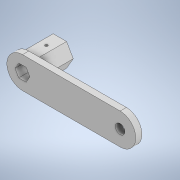
# Autodesk Inventor part: Acople_TransPot
Saved by Autodesk Inventor 2022 (Build 260153000, 153)
## iProperties
Created: 2022-02-22
Part Number: Acople_TransPot
Material: Generic
Document SubType Name: Modeling
Designer: katha
Density: 1 g/cm^3
Appearance: Default
Author: katha
Autodesk Inventor part; units mm, degrees
ref_plane "YZ Plane" through (0, 0, 0) normal (1, 0, 0) x (0, 1, 0)
ref_plane "XZ Plane" through (0, 0, 0) normal (0, 1, 0) x (-1, 0, 0)
ref_plane "Work Plane4" through (0, 0, 3) normal (0, 0, 1) x (1, 0, 0)
sketch "Sketch3" plane through (0, 0, 3) normal (0, 0, 1) x (1, 0, 0)
  circle A0 centre (47, 0) radius 2.3
  circle A1 centre (0, 0) radius 7.5 projected
  circle A2 centre (47, 0) radius 7.5
  line L0 (0, -7.5) -> (47, -7.5)
  line L1 (47, 0) -> (12.3969, 0) construction
  line L2 (0, 7.5) -> (47, 7.5)
  point P0 (0, 0)
  dimension "d13" = 15
  dimension "d5" = 4.6
  dimension "d14" = 47
  constraints: 6 end point, 3 horizontal, 2 symmetric about line, 1 centre point, 1 coincident, 5 other
  measures "d5" diameter of A0
  measures "d14" distance of L0.start L0.end
extrude "Extrusion5" add sketch "Sketch3" along normal blind 3
sketch "Sketch6" plane through (0, 0, 3) normal (0, 0, -1) x (-1, 0, 0)
  arc A0 (0, -7.5) -> (0, 7.5) centre (0, 0) ccw projected
  line L0 (0, 0) -> (3.1, 0) construction
  line L1 (0, 0) -> (1.55, 2.6847) construction
  line L2 (0, 0) -> (-1.55, 2.6847) construction
  line L3 (0, 0) -> (-3.1, 0) construction
  line L4 (0, 0) -> (-1.55, -2.6847) construction
  line L5 (0, 0) -> (1.55, -2.6847) construction
  line L6 (-1.55, 2.6847) -> (1.55, 2.6847) construction
  line L7 (1.55, 2.6847) -> (3.1, 0) construction
  line L8 (3.1, 0) -> (1.55, -2.6847) construction
  line L9 (1.55, -2.6847) -> (-1.55, -2.6847) construction
  line L10 (-1.55, -2.6847) -> (-3.1, 0) construction
  line L11 (-3.1, 0) -> (-1.55, 2.6847) construction
  line L12 (3.5619, 0) -> (1.7809, 3.0847)
  line L13 (1.7809, 3.0847) -> (-1.7809, 3.0847)
  line L14 (-1.7809, 3.0847) -> (-3.5619, 0)
  line L15 (-3.5619, 0) -> (-1.7809, -3.0847)
  line L16 (-1.7809, -3.0847) -> (1.7809, -3.0847)
  line L17 (1.7809, -3.0847) -> (3.5619, 0)
  line L18 (3.2243, 5.5847) -> (6.4486, 0)
  line L19 (6.4486, 0) -> (3.2243, -5.5847)
  line L20 (3.2243, -5.5847) -> (-3.2243, -5.5847)
  line L21 (-3.2243, -5.5847) -> (-6.4486, 0)
  line L22 (-6.4486, 0) -> (-3.2243, 5.5847)
  line L23 (-3.2243, 5.5847) -> (3.2243, 5.5847)
  point P0 (0, 0)
  dimension "d17" = 3.1
  dimension "d20" = 360
  dimension "d22" = 0.4
  dimension "d23" = 2.5
  constraints: 48 end point, 9 parallel, 2 coincident, 2 horizontal, 27 other
  measures "d17" distance of L0.start L0.end
  measures "d22" distance between parallel lines of L7 L12
  measures "d23" distance between parallel lines of L12 L18
extrude "Extrusion6" add sketch "Sketch6" along normal blind 15
sketch "Sketch7" plane through (0, 0, 3) normal (0, 0, -1) x (-1, 0, 0)
  line L0 (3.5619, 0) -> (1.7809, 3.0847) projected
  line L1 (1.7809, 3.0847) -> (-1.7809, 3.0847) projected
  line L2 (-1.7809, 3.0847) -> (-3.5619, 0) projected
  line L3 (-3.5619, 0) -> (-1.7809, -3.0847) projected
  line L4 (-1.7809, -3.0847) -> (1.7809, -3.0847) projected
  line L5 (1.7809, -3.0847) -> (3.5619, 0) projected
  point P0 (0, 0)
extrude "Extrusion7" cut sketch "Sketch7" against normal blind 15
sketch "Sketch8" plane through (-3.2243, 5.5847, 3) normal (0, 1, 0) x (1, 0, 0)
  line L0 (6.4486, 0) -> (0, 0) projected
  line L1 (6.4486, 0) -> (6.4486, 15) projected
  line L2 (0, 15) -> (6.4486, 15) projected
  line L3 (0, 0) -> (0, 15) projected
  line L4 (0, 0) -> (0, 15) projected
  line L5 (1.4434, 15) -> (5.0053, 15) projected
  line L6 (3.2243, 0) -> (3.2243, -3) projected
  line L7 (3.2243, 15) -> (3.2243, 0) construction
  circle A0 centre (3.2243, 8.5) radius 0.65
  line L8 (-4.2757, -3) -> (3.2243, -3) projected
  point P0 (3.2243, 3)
  dimension "d29" = 1.3
  dimension "d30" = 11.5
  constraints: 2 end point, 1 centre point, 1 midpoint, 1 point on line, 1 vertical
  measures "d29" diameter of A0
  measures "d30" distance from line of A0.centre L8
extrude "Extrusion8" cut sketch "Sketch8" against normal blind 15 contours A0
body "Solid1"
